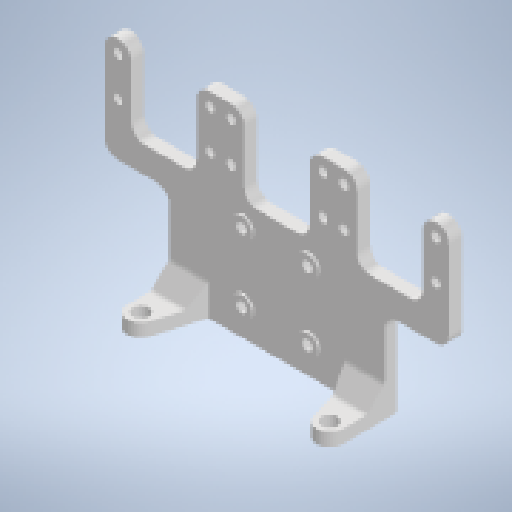
# Autodesk Inventor part: lacznik
Saved by Autodesk Inventor 2023 (Build 270158000, 158)
## iProperties
Created: 2024-05-16
Part Number: lacznik
Material: Ogólny
Document SubType Name: Modeling
Designer: kamil
Density: 1 g/cm^3
Appearance: Domyślna
Author: kamil
Autodesk Inventor part; units mm, degrees
ref_plane "YZ Plane" through (0, 0, 0) normal (1, 0, 0) x (0, 1, 0)
ref_plane "XZ Plane" through (0, 0, 0) normal (0, 1, 0) x (-1, 0, 0)
ref_plane "XY Plane" through (0, 0, 0) normal (0, 0, 1) x (1, 0, 0)
sketch "Szkic1" plane through (0, 0, 0) normal (0, 0, 1) x (1, 0, 0)
  circle A0 centre (-103.5, 7.875) radius 1.6 projected
  circle A1 centre (-103.5, -7.125) radius 1.6 projected
  circle A2 centre (-68.5, 7.875) radius 1.6 projected
  circle A3 centre (-60.5, 7.875) radius 1.6 projected
  circle A4 centre (-68.5, -7.125) radius 1.6 projected
  circle A5 centre (-60.5, -7.125) radius 1.6 projected
  circle A6 centre (-25.5, 7.875) radius 1.6 projected
  circle A7 centre (-25.5, -7.125) radius 1.6 projected
  circle A8 centre (-17.5, 7.875) radius 1.6 projected
  circle A9 centre (-17.5, -7.125) radius 1.6 projected
  circle A10 centre (17.5, 7.875) radius 1.6 projected
  circle A11 centre (17.5, -7.125) radius 1.6 projected
  line L0 (-108.5, 12.875) -> (-98.5, 12.875)
  line L1 (-98.5, 12.875) -> (-98.5, -17.125)
  line L2 (-98.5, -17.125) -> (-108.5, -17.125)
  line L3 (-108.5, -17.125) -> (-108.5, 12.875)
  line L4 (-73.5, 12.875) -> (-55.5, 12.875)
  line L5 (-55.5, 12.875) -> (-55.5, -17.125)
  line L6 (-55.5, -17.125) -> (-73.5, -17.125)
  line L7 (-73.5, -17.125) -> (-73.5, 12.875)
  line L8 (-30.5, 12.875) -> (-12.5, 12.875)
  line L9 (-12.5, 12.875) -> (-12.5, -17.125)
  line L10 (-12.5, -17.125) -> (-30.5, -17.125)
  line L11 (-30.5, -17.125) -> (-30.5, 12.875)
  line L12 (12.5, 12.875) -> (22.5, 12.875)
  line L13 (22.5, 12.875) -> (22.5, -17.125)
  line L14 (22.5, -17.125) -> (12.5, -17.125)
  line L15 (12.5, -17.125) -> (12.5, 12.875)
  circle A12 centre (-103.5, 7.875) radius 1.6 projected
  line L16 (-108.5, -17.125) -> (22.5, -17.125)
  line L17 (22.5, -17.125) -> (22.5, -27.125)
  line L18 (22.5, -27.125) -> (-108.5, -27.125)
  line L19 (-108.5, -27.125) -> (-108.5, -17.125)
  line L20 (-84, -62.125) -> (-2, -62.125)
  line L21 (-2, -62.125) -> (-2, -27.125)
  line L22 (-2, -27.125) -> (-84, -27.125)
  line L23 (-84, -27.125) -> (-84, -62.125)
  point P0 (0, 0)
  point P1 (22.5, -22.125)
  point P2 (22.5, -2.125)
  point P3 (-43, -27.125)
  point P4 (-43, -27.125)
  point P5 (-2, -27.125)
  dimension "d0" = 5
  dimension "d1" = 5
  dimension "d2" = 10
  dimension "d3" = 5
  dimension "d4" = 5
  dimension "d5" = 10
  dimension "d6" = 5
  dimension "d7" = 5
  dimension "d8" = 5
  dimension "d9" = 5
  dimension "d10" = 5
  dimension "d12" = 5
  dimension "d13" = 10
  dimension "d14" = 5
  dimension "d15" = 5
  dimension "d16" = 10
  dimension "d17" = 10
  dimension "d18" = 82
  dimension "d19" = 35
  constraints: 48 end point, 12 parallel, 6 horizontal, 6 perpendicular, 4 midpoint, 2 vertical alignment, 1 coincident, 1 horizontal alignment
  measures "d0" distance from line of L0 A0.centre
  measures "d1" distance from line of A0.centre L3
  measures "d2" distance from line of A1.centre L2
  measures "d3" distance from line of A0.centre L1
  measures "d4" distance from line of L4 A2.centre
  measures "d5" distance from line of L6 A4.centre
  measures "d6" distance from line of A2.centre L7
  measures "d7" distance from line of L5 A3.centre
  measures "d8" distance from line of A6.centre L8
  measures "d9" distance from line of L11 A6.centre
  measures "d10" distance from line of L9 A8.centre
  measures "d12" distance from line of A10.centre L12
  measures "d13" distance from line of L14 A11.centre
  measures "d14" distance from line of A11.centre L13
  measures "d15" distance from line of L15 A11.centre
  measures "d16" distance from line of L10 A9.centre
  measures "d17" distance of L16.end L17.end
  measures "d18" distance of L22.end L21.end
  measures "d19" distance of L21.end L20.end
extrude "Wyciągnięcie proste1" add sketch "Szkic1" along normal blind 5 contours A0 | A1 | A2 | A3 | A4 | A5 | A6 | A7 | A8 | A9 | A10 | A11 | L0 L1 L2 L3 | L2 L16 L6 L10 L14 L17 L18 L19 | L7 L4 L5 L6 | L18 L21 L20 L23 | L11 L8 L9 L10 | L14 L15 L12 L13
sketch "Szkic2" plane through (-84, -62.125, 0) normal (0, -1, 0) x (1, 0, 0)
  line L0 (0, 5) -> (82, 5) projected
  circle A0 centre (77, 20.9) radius 2 projected
  circle A1 centre (5, 20.9) radius 2 projected
  line L1 (82, 25.4) -> (82, 0.4) projected
  line L2 (0, 0.4) -> (0, 25.4) projected
  circle A2 centre (77, 20.9) radius 5
  circle A3 centre (5, 20.9) radius 5
  line L3 (67, 5) -> (72.2116, 22.3392)
  line L4 (15, 5) -> (9.7884, 22.3392)
  point P0 (84, 0)
  point P1 (0, 20.9)
  point P2 (82, 20.9)
  dimension "d22" = 15
  dimension "d23" = 15
  constraints: 4 end point, 2 coincident, 2 point on line, 2 vertical, 8 other
  measures "d22" distance of L3.start L0.end
  measures "d23" distance of L0.start L4.start
extrude "Wyciągnięcie proste2" add sketch "Szkic2" against normal blind 5
chamfer "Faza1" distance 7 angle 45 2 edges at (-76.5, -57.125, 5) (-9.5, -57.125, 5)
fillet "Zaokrąglenie1" radius 2 4 edges at (-77.552, -57.125, 12) (-8.448, -57.125, 12) (-9.5, -50.125, 5) (-76.5, -50.125, 5)
fillet "Zaokrąglenie2" radius 5 18 edges at (-2, -27.125, 2.5) (22.5, -27.125, 2.5) (12.5, -17.125, 2.5) (12.5, 12.875, 2.5) (22.5, 12.875, 2.5) (-12.5, -17.125, 2.5) (-12.5, 12.875, 2.5) (-30.5, 12.875, 2.5) (-30.5, -17.125, 2.5) (-55.5, -17.125, 2.5) (-55.5, 12.875, 2.5) (-98.5, -17.125, 2.5) (-108.5, 12.875, 2.5) (-98.5, 12.875, 2.5) (-73.5, -17.125, 2.5) (-73.5, 12.875, 2.5) (-108.5, -27.125, 2.5) (-84, -27.125, 2.5)
sketch "Szkic4" plane through (0, 0, 5) normal (0, 0, 1) x (1, 0, 0)
  circle A0 centre (-30.5, -53.125) radius 1.6 projected
  circle A1 centre (-55.5, -53.125) radius 1.6 projected
  circle A2 centre (-55.5, -27.125) radius 1.6 projected
  circle A3 centre (-30.5, -27.125) radius 1.6 projected
  circle A4 centre (-30.5, -53.125) radius 4
  circle A5 centre (-55.5, -53.125) radius 4
  circle A6 centre (-55.5, -27.125) radius 4
  circle A7 centre (-30.5, -27.125) radius 4
  point P0 (0, 0)
  dimension "d38" = 8
  dimension "d39" = 8
  dimension "d40" = 8
  dimension "d41" = 8
  constraints: 4 centre point, 4 coincident
  measures "d38" diameter of A4
  measures "d39" diameter of A5
  measures "d40" diameter of A6
  measures "d41" diameter of A7
ref_plane "Płaszczyzna konstrukcyjna1" through (-67.5, -57.125, 6) normal (0, 0, -1) x (0, 1, 0)
extrude "Wyciągnięcie proste3" add sketch "Szkic4" along normal up to surface (1 mm away) contours A0 | A1 | A2 | A3 | A4 | A5 | A6 | A7
sketch "Szkic5" plane through (-30.5, -27.125, 6) normal (0, 0, 1) x (1, 0, 0)
  circle A0 centre (0, 0) radius 1.6 projected
  circle A1 centre (-25, 0) radius 1.6 projected
  circle A2 centre (0, -26) radius 1.6 projected
  circle A3 centre (-25, -26) radius 1.6 projected
  point P0 (30.5, 27.125)
hole "Otwór2" at (-30.5, -53.125, 6) at (-30.5, -27.125, 6) at (-55.5, -53.125, 6) at (-55.5, -27.125, 6) direction (0, 0, -1) diameter 3.5 depth 10 counterbore diameter 4 counterbore depth 5
fillet "Zaokrąglenie3" [suppressed]
sketch "Szkic6" plane through (0, 0, 0) normal (0, 0, -1) x (-1, 0, 0)
  circle A0 centre (-17.5, -7.125) radius 1.6 projected
  circle A1 centre (-17.5, 7.875) radius 1.6 projected
  circle A2 centre (17.5, 7.875) radius 1.6 projected
  circle A3 centre (17.5, -7.125) radius 1.6 projected
  circle A4 centre (25.5, 7.875) radius 1.6 projected
  circle A5 centre (25.5, -7.125) radius 1.6 projected
  circle A6 centre (60.5, 7.875) radius 1.6 projected
  circle A7 centre (60.5, -7.125) radius 1.6 projected
  circle A8 centre (68.5, 7.875) radius 1.6 projected
  circle A9 centre (68.5, -7.125) radius 1.6 projected
  circle A10 centre (103.5, 7.875) radius 1.6 projected
  circle A11 centre (103.5, -7.125) radius 1.6 projected
  point P0 (0, 0)
hole "Otwór3" at (17.5, -7.125, 0) at (17.5, 7.875, 0) at (-17.5, 7.875, 0) at (-17.5, -7.125, 0) at (-25.5, -7.125, 0) at (-25.5, 7.875, 0) at (-60.5, 7.875, 0) at (-60.5, -7.125, 0) at (-68.5, 7.875, 0) at (-68.5, -7.125, 0) at (-103.5, -7.125, 0) at (-103.5, 7.875, 0) direction (0, 0, 1) diameter 3.5 depth 10 counterbore diameter 4 counterbore depth 4
sketch "Szkic7" plane through (-84, -57.125, 0) normal (0, 1, 0) x (1, 0, 0)
  circle A0 centre (77, -20.9) radius 2 projected
  circle A1 centre (5, -20.9) radius 2 projected
  point P0 (84, 0)
extrude "Wyciągnięcie proste4" add sketch "Szkic7" against normal up to surface (5 mm away)
sketch "Szkic8" plane through (-84, -57.125, 0) normal (0, 1, 0) x (1, 0, 0)
  line L0 (69.353, -12.8284) -> (82, -12.8284) projected
  line L1 (69.353, -12.8284) -> (72.2116, -22.3392) projected
  arc A0 (72.2116, -22.3392) -> (82, -20.9) centre (77, -20.9) ccw projected
  line L2 (82, -20.9) -> (82, -12.8284) projected
  line L3 (0, -12.8284) -> (12.647, -12.8284) projected
  line L4 (0, -12.8284) -> (0, -20.9) projected
  arc A1 (0, -20.9) -> (9.7884, -22.3392) centre (5, -20.9) ccw projected
  line L5 (9.7884, -22.3392) -> (12.647, -12.8284) projected
  point P0 (84, 0)
hole "Otwór4" at (-7, -57.125, 20.9) at (-79, -57.125, 20.9) direction (0, -1, 0) diameter 3.3 depth 10 counterbore diameter 6 counterbore depth 4
sketch "Szkic9" plane through (0, 0, 5) normal (0, 0, 1) x (1, 0, 0)
  circle A0 centre (-12.275, -34.7108) radius 1.75 projected
  circle A1 centre (-73.725, -34.7108) radius 1.75 projected
  point P0 (0, 0)
hole "Otwór5" at (-12.275, -34.7108, 5) at (-73.725, -34.7108, 5) direction (0, 0, -1) diameter 3.5 end through all counterbore diameter 4 counterbore depth 4
sketch "Szkic10" plane through (0, 0, 5) normal (0, 0, 1) x (1, 0, 0)
  circle A0 centre (17.5, -7.125) radius 1.75 projected
  circle A1 centre (17.5, 7.875) radius 1.75 projected
  circle A2 centre (-103.5, -7.125) radius 1.75 projected
  point P0 (0, 0)
  point P1 (17.5, -19.125)
  point P2 (-103.5, -19.125)
  dimension "d75" = 12
  dimension "d76" = 12
  constraints: 2 vertical alignment
  measures "d75" distance of point (17.5, -19.125) A0.centre
  measures "d76" distance of A2.centre point (-103.5, -19.125)
hole "Otwór6" at (17.5, -19.125, 5) at (-103.5, -19.125, 5) direction (0, 0, -1) diameter 3.5 end through all counterbore diameter 4 counterbore depth 4
